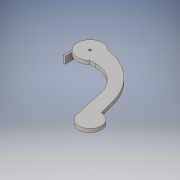
# Autodesk Inventor part: Part4
Saved by Autodesk Inventor 2016 (Build 200138000, 138)
## iProperties
Created: 2016-01-12
Part Number: Part4
Material: Generic
Document SubType Name: Modeling
Designer: cemer
Density: 1 g/cm^3
Appearance: Default
Author: cemer
Autodesk Inventor part; units mm, degrees
ref_plane "YZ Plane" through (0, 0, 0) normal (1, 0, 0) x (0, 1, 0)
ref_plane "XZ Plane" through (0, 0, 0) normal (0, 1, 0) x (-1, 0, 0)
ref_plane "XY Plane" through (0, 0, 0) normal (0, 0, 1) x (1, 0, 0)
sketch "Sketch1" plane through (0, 0, 0) normal (0, 1, 0) x (-1, 0, 0)
  circle A0 centre (0, 0) radius 11.43
  circle A1 centre (0, 0) radius 9.525
  dimension "d0" = 22.86
  dimension "d1" = 19.05
  constraints: 2 centre point, 2 coincident
  measures "d0" diameter of A0
  measures "d1" diameter of A1
extrude "Extrusion1" add sketch "Sketch1" along normal blind 6.35
sketch "Sketch2" plane through (0, 6.35, 0) normal (0, 1, 0) x (1, 0, 0)
  circle A0 centre (0, 0) radius 11.43
  constraints: 1 centre point, 1 coincident
extrude "Extrusion2" add sketch "Sketch2" along normal blind 3.175
sketch "Sketch3" plane through (0, 9.525, 0) normal (0, 1, 0) x (1, 0, 0)
  circle A0 centre (0, 0) radius 1.1
  dimension "d6" = 2.2
  constraints: 1 centre point, 1 coincident
  measures "d6" diameter of A0
extrude "Extrusion3" cut sketch "Sketch3" against normal blind 7.9375
sketch "Sketch6" plane through (0, 0, 0) normal (0, -1, 0) x (1, 0, 0)
  line L0 (-16.0948, 0) -> (0, 0)
  line L1 (0, 0) -> (0, -15.3841)
  line L2 (0, -15.3841) -> (-16.0948, -15.3841)
  line L3 (-16.0948, -15.3841) -> (-16.0948, 0)
  line L4 (-16.0948, 14.6504) -> (12.3807, 14.6504)
  line L5 (12.3807, 14.6504) -> (12.3807, -15.3841)
  line L6 (12.3807, -15.3841) -> (-16.0948, -15.3841)
  line L7 (-16.0948, -15.3841) -> (-16.0948, 14.6504)
  constraints: 16 end point, 4 parallel, 2 horizontal, 2 perpendicular
extrude "Extrusion6" cut sketch "Sketch6" against normal blind 6.35 contours L7 L4 L5 L6 L1 L0
sketch "Sketch7" plane through (0, 0, -9.525) normal (1, 0, 0) x (0, 0, -1)
  line L0 (1.905, 6.35) -> (-20.955, 6.35) projected
  line L1 (1.905, 6.35) -> (0, 6.35)
  line L2 (0, 6.35) -> (0, 0)
  line L3 (0, 0) -> (1.905, 0)
  line L4 (1.905, 0) -> (1.905, 6.35)
  point P0 (-9.525, 0)
  point P1 (-9.525, 6.35)
  constraints: 8 end point, 2 parallel, 1 horizontal, 1 perpendicular
extrude "Extrusion7" add sketch "Sketch7" along normal blind 11.43
sketch "Sketch16" plane through (0, 0, 0) normal (0, -1, 0) x (1, 0, 0)
  point P0 (0, 0)
sketch "Sketch17" plane through (-11.43, 0, 0) normal (0, 0, 1) x (1, 0, 0)
  line L0 (0, 0) -> (0, 6.35) projected
  line L1 (0, 6.35) -> (1.9041, 6.35)
  line L2 (1.9041, 6.35) -> (1.9041, 0)
  line L3 (1.9041, 0) -> (0, 0)
  line L4 (0, 0) -> (0, 6.35)
  point P0 (11.43, 0)
  constraints: 8 end point, 2 parallel, 1 horizontal, 1 perpendicular
extrude "Extrusion16" add sketch "Sketch17" along normal blind 12.7
sketch "Sketch18" plane through (0, 6.35, 0) normal (0, -1, 0) x (1, 0, 0)
  circle A0 centre (0, 0) radius 1.1 projected
  line L0 (0, 0) -> (-18.4871, -7.6576)
  line L1 (0, 0) -> (20.0102, 0) construction
  line L2 (-18.4871, -7.6576) -> (1.1, -41.4972)
  line L3 (1.1, -41.4972) -> (21.3747, 0)
  line L4 (21.3747, 0) -> (0, 0)
  dimension "d61" = 157.5
  constraints: 10 end point, 2 horizontal, 1 equal length
  measures "d61" angle of L0 L1
extrude "Extrusion17" cut sketch "Sketch18" along normal blind 25.4 contours L4 L3 L2 L0 A0 | A0 L0 L4 picked at (-0.5236, -0.5052)
sketch "Sketch21" plane through (0, 9.525, 0) normal (0, 1, 0) x (1, 0, 0)
  line L0 (0, 0) -> (76.2, 0) construction
  circle A0 centre (0, 0) radius 11.43 projected
  line L1 (8.0168, -8.1472) -> (33.4168, -8.1472)
  line L2 (8.0168, -8.1472) -> (33.4168, -8.1472) construction
  circle A1 centre (53.8815, -53.8815) radius 10.16
  line L3 (33.4168, -8.1472) -> (46.6973, -46.6973)
  line L4 (8.0822, 8.0822) -> (38.5622, 8.0822)
  line L5 (53.8815, -53.8815) -> (61.0657, -46.6973)
  line L6 (53.8815, -53.8815) -> (64.0415, -53.8815) construction
  line L7 (61.0657, -46.6973) -> (38.5622, 8.0822)
  line L8 (0, 0) -> (8.0168, -8.1472)
  line L9 (46.6973, -46.6973) -> (53.8815, -53.8815)
  line L10 (8.0168, 8.1472) -> (8.0168, -8.1472)
  dimension "d85" = 25.4
  dimension "d86" = 0
  dimension "d87" = 20.32
  dimension "d88" = 30.48
  dimension "d89" = 45
  constraints: 22 end point, 5 horizontal, 5 point on circle, 2 equal length, 1 centre point, 1 coincident, 1 vertical
  measures "d85" distance of L1.start L1.end
  measures "d86" distance between parallel lines of L1 L2
  measures "d87" diameter of A1
  measures "d88" distance of L4.start L4.end
  measures "d89" angle of L6 L5
extrude "Extrusion20" add sketch "Sketch21" against normal blind 3.175 contours L5 L9 A1 | A1 L9 L5
sketch "Sketch22" plane through (0, 9.525, 0) normal (0, 1, 0) x (1, 0, 0)
  circle A0 centre (0, 0) radius 1.1 projected
  line L0 (0, 0) -> (8.0822, 8.0822)
  circle A1 centre (0, 0) radius 11.43 projected
  line L1 (0, 0) -> (11.43, 0) construction
  line L2 (8.0822, 8.0822) -> (39.8322, 8.0822)
  line L3 (39.8322, 8.0822) -> (53.8815, -43.7215)
  circle A2 centre (53.8815, -53.8815) radius 10.16 projected
  line L4 (0, 0) -> (8.0822, -8.0822)
  line L5 (8.0822, -8.0822) -> (33.4822, -8.0822)
  line L6 (33.4822, -8.0822) -> (43.7215, -53.8815)
  line L7 (53.8815, -43.7215) -> (43.7215, -53.8815)
  dimension "d92" = 45
  dimension "d93" = 31.75
  dimension "d94" = 25.4
  constraints: 16 end point, 5 point on circle, 2 horizontal, 1 equal length, 1 parallel, 1 perpendicular, 1 point on line
  measures "d92" angle of L1 L0
  measures "d93" distance of L0.end L2.end
  measures "d94" distance of L4.end L5.end
extrude "Extrusion21" add sketch "Sketch22" against normal blind 3.175 contours L2 L3 A2 L6 L5 A1
fillet "Fillet6" radius 25.4 1 edges at (33.4822, 7.9375, 8.0822)
fillet "Fillet7" radius 50.8 1 edges at (39.8322, 7.9375, -8.0822)
body "Solid1"
